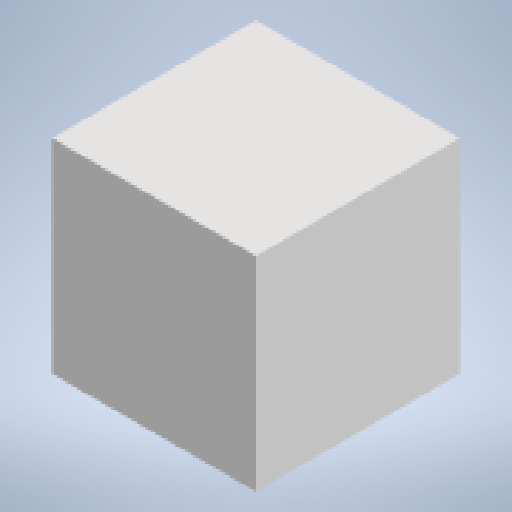
# Autodesk Inventor part: load
Saved by Autodesk Inventor 2024.3 (Build 283343010, 343A)
## iProperties
Created: 2025-09-22
Part Number: load
Material: 一般
Document SubType Name: Modeling
Designer: kshau
Mass: 1500 g
Surface Area: 150 cm^2
Volume: 125 cm^3
Density: 12 g/cm^3
Appearance: 既定
Author: kshau
Autodesk Inventor part; units mm, degrees
ref_plane "YZ Plane" through (0, 0, 0) normal (1, 0, 0) x (0, 1, 0)
ref_plane "XZ Plane" through (0, 0, 0) normal (0, 1, 0) x (-1, 0, 0)
ref_plane "XY Plane" through (0, 0, 0) normal (0, 0, 1) x (1, 0, 0)
sketch "スケッチ1" plane through (0, 0, 0) normal (0, 1, 0) x (-1, 0, 0)
  line L0 (0, 0) -> (50, 0)
  line L1 (50, 0) -> (50, -50)
  line L2 (50, -50) -> (0, -50)
  line L3 (0, -50) -> (0, 0)
  dimension "d0" = 50
  dimension "d1" = 50
  constraints: 8 end point, 2 parallel, 1 horizontal, 1 perpendicular
  measures "d0" distance of L1.end L2.end
  measures "d1" distance of L0.end L1.end
extrude "押し出し1" add sketch "スケッチ1" along normal blind 50
